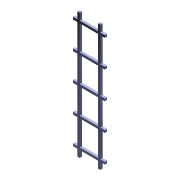
# Autodesk Inventor part: Rail zone
Saved by Autodesk Inventor 2015 (Build 190159000, 159)
## iProperties
Created: 2015-03-07
Part Number: Rail zone
Material: Generic
Document SubType Name: Modeling
Designer: Vukica
Density: 1 g/cm^3
Appearance: Chrome - Polished Blue
Author: Vukica
Autodesk Inventor part; units mm, degrees
ref_plane "YZ Plane" through (0, 0, 0) normal (1, 0, 0) x (0, 1, 0)
ref_plane "XZ Plane" through (0, 0, 0) normal (0, 1, 0) x (-1, 0, 0)
ref_plane "XY Plane" through (0, 0, 0) normal (0, 0, 1) x (1, 0, 0)
sketch "Sketch1" plane through (0, 0, 0) normal (0, 0, 1) x (1, 0, 0)
  line L0 (-127, 698.5) -> (-101.6, 698.5)
  line L1 (-101.6, 698.5) -> (-101.6, -698.5)
  line L2 (-101.6, -698.5) -> (-127, -698.5)
  line L3 (-127, -698.5) -> (-127, 698.5)
  line L4 (101.6, 698.5) -> (127, 698.5)
  line L5 (127, 698.5) -> (127, -698.5)
  line L6 (127, -698.5) -> (101.6, -698.5)
  line L7 (101.6, -698.5) -> (101.6, 698.5)
  line L8 (0, 0) -> (0, 143.5331) construction
  line L9 (0, 0) -> (-211.7363, 0) construction
  dimension "d0" = 25.4
  dimension "d1" = 1397
  dimension "d2" = 203.2
  constraints: 20 end point, 4 parallel, 3 horizontal, 2 equal length, 2 perpendicular, 2 vertical, 1 collinear, 1 horizontal alignment, 2 other
  measures "d0" distance of L0.start L0.end
  measures "d1" distance of L2.end L0.start
  measures "d2" distance between parallel lines of L1 L7
extrude "Extrusion1" add sketch "Sketch1" along normal blind 25.4
sketch "Sketch2" plane through (0, 0, 25.4) normal (0, 0, 1) x (1, 0, 0)
  line L0 (-177.8, 622.3) -> (177.8, 622.3)
  line L1 (177.8, 622.3) -> (177.8, 596.9)
  line L2 (177.8, 596.9) -> (-177.8, 596.9)
  line L3 (-177.8, 596.9) -> (-177.8, 622.3)
  line L4 (0, 0) -> (0, 410.334) construction
  line L5 (127, 698.5) -> (101.6, 698.5) construction
  dimension "d5" = 25.4
  dimension "d6" = 355.6
  dimension "d7" = 76.2
  constraints: 10 end point, 2 parallel, 2 vertical, 1 horizontal, 1 perpendicular, 1 other
  measures "d5" distance of L0.end L1.end
  measures "d6" distance of L0.start L0.end
  measures "d7" distance between parallel lines of L0 L5
extrude "Extrusion2" add sketch "Sketch2" against normal blind 25.4
pattern_linear "Rectangular Pattern1" count 5 spacing 304.8 along (0, -1, 0) of "Extrusion2"
body "Solid1"
